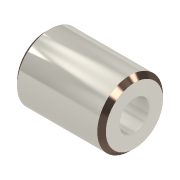
# Autodesk Inventor part: Roller
Saved by Autodesk Inventor 2022.2 (Build 262287010, 287A)
## iProperties
Created: 2022-12-22
Part Number: Roller
Material: Steel
Document SubType Name: Modeling
Designer: User
Density: 7.85 g/cm^3
Appearance: Gunmetal - Antique Polished
Author: User
Autodesk Inventor part; units mm, degrees
ref_plane "YZ Plane" through (0, 0, 0) normal (1, 0, 0) x (0, 1, 0)
ref_plane "XZ Plane" through (0, 0, 0) normal (0, 1, 0) x (-1, 0, 0)
ref_plane "XY Plane" through (0, 0, 0) normal (0, 0, 1) x (1, 0, 0)
sketch "Sketch1" plane through (0, 0, 0) normal (0, 0, 1) x (1, 0, 0)
  line L0 (-5, 3.7) -> (5, 3.7)
  line L1 (5, 3.7) -> (5, 1.7)
  line L2 (5, 0) -> (-5, 0)
  line L3 (-5, 0) -> (-5, 1.7) construction
  line L4 (-5, 1.7) -> (5, 1.7)
  line L5 (-5, 1.7) -> (-5, 3.7)
  line L6 (5, 1.7) -> (5, 0) construction
  point P0 (0, 0)
  point P1 (0, 0)
  dimension "d0" = 7.4
  dimension "d1" = 3.4
  dimension "d2" = 10
  constraints: 14 end point, 5 parallel, 4 perpendicular, 1 coincident, 1 horizontal, 1 midpoint
  measures "d0" diameter of L0 L2
  measures "d1" diameter of L4 L2
  measures "d2" distance of L0.start L0.end
revolve "Revolution1" add sketch "Sketch1" angle 360 about axis through (5, 0, 0) along (-1, 0, 0)
chamfer "Chamfer1" distance 0.5 angle 45 2 edges at (5, -3.7, 0) (-5, -3.7, 0)
body "Solid1"
